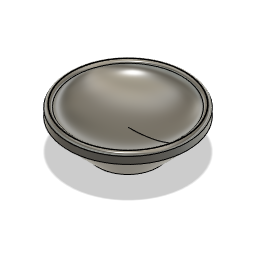
Concave_Topper (Autodesk Fusion 360 design; units mm, degrees)
Autodesk Fusion 360 part; units mm, degrees
note: some values were not read from the file. Set by a fixed rule: which sketch regions a step uses; which face or edge a step refers to.
sketch "Concave Profile" plane through (0, 0, 0) normal (0, 0, 1) x (1, 0, 0)
  line L0 (-30, 10) -> (-30, 20)
  line L1 (-30, 20) -> (-27, 20)
  line L2 (30, 10) -> (30, 20)
  line L3 (30, 20) -> (27, 20)
  line L4 (0, 0) -> (0, 10)
  line L5 (30, 10) -> (-30, 10) construction
  line L6 (-30, 10) -> (-30, 0)
  line L7 (30, 10) -> (30, 0)
  line L8 (-30, 0) -> (30, 0)
  line L9 (15, 0) -> (30, 15)
  ellipse E0 centre (0, 20) end of major axis (27, 20) minor radius 10
  line L10 (-27, 20) -> (27, 20)
  line L11 (0, 10) -> (0, 30)
  dimension "d7" = 10
  dimension "d8" = 10
  dimension "d10" = 3
  dimension "d32" = 45
  dimension "d34" = 60
  dimension "d40" = 15
  constraint perpendicular L0 L1
  constraint perpendicular L2 L3
  constraint coincident L4.start origin
  constraint equal L0 L2
  constraint perpendicular L4 L5
  constraint coincident L2.start L5.start
  constraint coincident L0.start L5.end
  constraint perpendicular L7 L8
  constraint midpoint L4.start L8
  constraint perpendicular L6 L8
  constraint parallel L2 L7
  constraint parallel L0 L6
  constraint equal L6 L7
  constraint coincident L8 L9.start
  constraint coincident E0 L1.end
  constraint coincident L3.end E0
  constraint coincident E0 L4.end
  constraint coincident E0 L11.end
  constraint collinear L1 L10
  constraint coincident L4.end L11.start
  constraint horizontal L8
  constraint coincident L5 L4.end
  constraint coincident L7 L9.end
  measures "d7" distance of L2.start L2.end
  measures "d8" distance of L7.end L2.start
  measures "d10" distance of L2.end L3.end
  measures "d32" angle of L8 L9
  measures "d34" distance of L0.end L2.end
  measures "d40" distance of L4.start L9.start
revolve "Revolve1" add sketch "Concave Profile" angle 360 about axis through (0, 0, 0) along (0, 1, 0) contours L2 L3 L4 L8 L9 E0
sketch "Thread Bore" plane through (0, 0, 0) normal (0, -1, 0) x (1, 0, 0)
  circle A0 centre (0, 0) radius 14
  circle A1 centre (0, 0) radius 30
  circle A2 centre (0, 0) radius 15
  dimension "d14" = 28
  constraint coincident A0.centre A1.centre
  measures "d14" diameter of A0
extrude "Extrude2" cut sketch "Thread Bore" against normal blind 6 contours A0
sketch "Collet Hole" plane through (0, 6, 0) normal (0, -1, 0) x (1, 0, 0)
  circle A0 centre (0, 0) radius 14
  circle A1 centre (0, 0) radius 9
  dimension "d17" = 18
  constraint coincident A0.centre A1.centre
  measures "d17" diameter of A1
extrude "Extrude3" cut sketch "Collet Hole" against normal blind 3 contours A1
sketch "Collet Interface" plane through (0, 0, 0) normal (0, 0, 1) x (1, 0, 0)
  line L0 (9, 9) -> (-9, 9)
  line L1 (9, 6) -> (-9, 6)
  line L2 (9, 6) -> (7.6706, 9)
  line L3 (9, 9) -> (9, 6)
  line L4 (0, 9) -> (0, 6)
  dimension "d20" = 66.1
  constraint coincident L1.start L2.start
  constraint coincident L0 L2.end
  constraint coincident L0.start L3.start
  constraint midpoint L0 L4.start
  constraint midpoint L1 L4.end
  measures "d20" angle of L0 L2
revolve "Revolve2" add sketch "Collet Interface" angle 360 about axis through (0, 9, 0) along (0, -1, 0) contours L0 L2 L3
sketch "Unsupported Hole" plane through (0, 6, 0) normal (0, -1, 0) x (1, 0, 0)
  circle A0 centre (0, 0) radius 9
  circle A1 centre (0, 0) radius 14
  line L0 (-13.2288, 9) -> (13.2288, 9)
  line L1 (9, 13.2288) -> (9, -13.2288)
  line L2 (13.2288, -9) -> (-13.2288, -9)
  line L3 (-9, -13.2288) -> (-9, 13.2288)
  circle A2 centre (0, 0) radius 16
  dimension "d37" = 32
  constraint horizontal L0
  constraint perpendicular L0 L1
  constraint perpendicular L1 L2
  constraint perpendicular L2 L3
  constraint tangent A0 L0
  constraint tangent A0 L3
  constraint tangent A0 L2
  constraint tangent A0 L1
  constraint concentric A0 A2
  constraint coincident L1.start A2
  constraint coincident L0.end A2
  constraint coincident L2.start A2
  constraint coincident L1.end A2
  constraint coincident L3.start A2
  constraint coincident L0.start A2
  constraint coincident L2.end A2
  constraint coincident L3.end A2
  measures "d37" diameter of A2
extrude "Extrude4" cut sketch "Unsupported Hole" against normal blind 0.4 contours A0 | A0 L1 L2 | A0 L0 L1 | A0 L0 L3 | A0 L2 L3
extrude "Extrude5" cut sketch "Unsupported Hole" against normal blind 0.2 contours A1 L0 L1 L2 | A1 L0 L2 L3 | A1 L0 L2 A2 | A1 L0 L2 A2
thread "Thread1" "ISO Metric profile 28.0 M28x2 6H" major diameter 28.2565 minor diameter 26.0224 pitch 2 angle 60 modelled right hand crest width 0.5434 on face at (0, 2, 14) crest through (13.0112, 0.5, 0)
chamfer "Chamfer2" distance 0.4 angle 45 1 edges at (-8.2257, 6.4, -3.1904)
fillet "Fillet1" radius 1.5 1 edges at (-27.9698, 20, -10.8485)
fillet "Fillet1" radius 1.5 1 edges at (-25.1728, 20, -9.7636)
extrude "Extrude6" add 2 faces at (13.1114, 6, 7.3172) (-13.1114, 6, 7.3172) along direction (0, 1, 0) blind 0.4
equation "Diameter = 60 mm" comment "Minimum 50mm"
equation "Depth = 10 mm" comment "Minimum 1mm"
equation "d7 = Depth"
equation "d10 = Rim_Width"
equation "Rim_Width = 3 mm" comment "Minimum 1mm"
equation "d28 = Rim_Width / 2"
equation "d34 = Diameter"
equation "d36 = Rim_Width / 2"
named bodies: "Concave_Topper"
